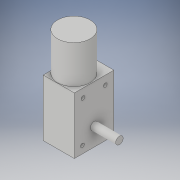
# Autodesk Inventor part: motor
Saved by Autodesk Inventor 2019 (Build 230136000, 136)
## iProperties
Created: 2018-09-07
Part Number: motor
Material: Generic
Document SubType Name: Modeling
Designer: mspet
Density: 1 g/cm^3
Appearance: Default
Author: mspet
Autodesk Inventor part; units mm, degrees
ref_plane "YZ Plane" through (0, 0, 0) normal (1, 0, 0) x (0, 1, 0)
ref_plane "XZ Plane" through (0, 0, 0) normal (0, 1, 0) x (-1, 0, 0)
ref_plane "XY Plane" through (0, 0, 0) normal (0, 0, 1) x (1, 0, 0)
sketch "Sketch1" plane through (0, 0, 0) normal (1, 0, 0) x (0, 1, 0)
  line L0 (0, 0) -> (46, 0)
  line L1 (46, 0) -> (46, -32)
  line L2 (46, -32) -> (0, -32)
  line L3 (0, -32) -> (0, 0)
  dimension "d0" = 46
  dimension "d1" = 32
  constraints: 8 end point, 2 parallel, 1 horizontal, 1 perpendicular
  measures "d0" distance of L1.end L2.end
  measures "d1" distance of L0.end L1.end
extrude "Extrusion1" add sketch "Sketch1" along normal blind 25.2
sketch "Sketch3" plane through (0, 46, 0) normal (0, 1, 0) x (1, 0, 0)
  circle A0 centre (11.23, 13.585) radius 13.2
  line L0 (25.2, 32) -> (25.2, 0) projected
  line L1 (0, 32) -> (25.2, 32) projected
  point P0 (0, 0)
  dimension "d4" = 26.4
  dimension "d5" = 13.97
  dimension "d6" = 18.415
  constraints: 1 centre point
  measures "d4" diameter of A0
  measures "d5" distance from line of L0 A0.centre
  measures "d6" distance from line of L1 A0.centre
extrude "Extrusion2" add sketch "Sketch3" along normal blind 30.8
sketch "Sketch4" plane through (25.2, 0, 0) normal (1, 0, 0) x (0, 0, -1)
  circle A0 centre (7, 39) radius 1.5
  circle A1 centre (25, 39) radius 1.5
  circle A2 centre (6.5, 6) radius 1.5
  circle A3 centre (24.5, 6) radius 1.5
  line L0 (32, 46) -> (0, 46) projected
  line L1 (32, 0) -> (32, 46) projected
  point P0 (0, 0)
  dimension "d9" = 3
  dimension "d10" = 3
  dimension "d11" = 3
  dimension "d12" = 3
  dimension "d13" = 7
  dimension "d14" = 7
  dimension "d15" = 18
  dimension "d16" = 33
  dimension "d17" = 33
  dimension "d18" = 18
  dimension "d19" = 7
  dimension "d20" = 7.5
  constraints: 4 centre point
  measures "d9" diameter of A1
  measures "d10" diameter of A0
  measures "d11" diameter of A3
  measures "d12" diameter of A2
  measures "d13" distance from line of L0 A0.centre
  measures "d14" distance from line of L0 A1.centre
  measures "d15" distance of A1.centre A0.centre
  measures "d16" vertical distance of A2.centre A0.centre
  measures "d17" vertical distance of A1.centre A3.centre
  measures "d18" distance of A2.centre A3.centre
  measures "d19" distance from line of L1 A1.centre
  measures "d20" distance from line of L1 A3.centre
extrude "Extrusion3" cut sketch "Sketch4" against normal blind 5
sketch "Sketch5" plane through (25.2, 0, 0) normal (1, 0, 0) x (0, 0, -1)
  circle A0 centre (15.998, 15) radius 3
  line L0 (32, 0) -> (32, 46) projected
  line L1 (0, 0) -> (32, 0) projected
  dimension "d23" = 6
  dimension "d24" = 16.002
  dimension "d25" = 15
  constraints: 1 centre point
  measures "d23" diameter of A0
  measures "d24" distance from line of L0 A0.centre
  measures "d25" distance from line of L1 A0.centre
extrude "Extrusion4" add sketch "Sketch5" along normal blind 20.5
body "Solid1"
